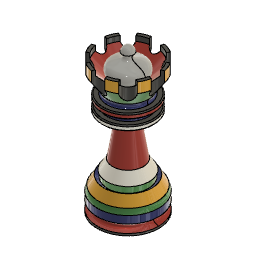
IRFAN NAUFAL CHESSPIECE EA v1 (Autodesk Fusion 360 design; units mm, degrees)
Autodesk Fusion 360 part; units mm, degrees
sketch "Sketch1" plane through (0, 0, 0) normal (0, 1, 0) x (1, 0, 0)
  line L0 (0, 0) -> (0, -140.5)
  line L1 (0, 0) -> (30, 0)
  line L2 (20.255, -85) -> (24.255, -85)
  line L3 (25.255, -86) -> (25.255, -89)
  line L4 (24.255, -90) -> (20.255, -90)
  line L5 (20.255, -90) -> (20.255, -95)
  line L6 (20.255, -95) -> (24.255, -95)
  line L7 (25.255, -96) -> (25.255, -99)
  line L8 (24.255, -100) -> (20.255, -100)
  line L9 (15, -45) -> (10, -75)
  spline S0 degree 5 poles (10, -75) (10.0092, -75.3857) (10.0449, -76.1408) (10.1499, -77.2245) (10.3948, -78.5701) (10.8875, -80.0753) (11.583, -81.3881) (12.4976, -82.4932) (13.6392, -83.3832) (14.9977, -84.0674) (16.5565, -84.5619) (17.9504, -84.8182) (19.0731, -84.9371) (19.8554, -84.9844) (20.255, -85) knots 0 0 0 0 0 0 0.1 0.2 0.3 0.4 0.5 0.6 0.7 0.8 0.9 1 1 1 1 1 1
  line L10 (20.255, -104.758) -> (30, -120)
  line L11 (30, -120) -> (30, -130)
  line L12 (30, -130) -> (27, -130)
  line L13 (27, -130) -> (27, -125)
  line L14 (27, -125) -> (13.4752, -111.6935)
  spline S1 degree 5 poles (20.255, -100) (20.1529, -100.0131) (19.9584, -100.047) (19.6954, -100.1209) (19.4032, -100.2666) (19.1413, -100.5318) (18.9896, -100.8856) (18.9526, -101.3317) (19.0262, -101.8667) (19.2009, -102.4829) (19.4662, -103.172) (19.7438, -103.776) (19.9863, -104.2565) (20.163, -104.5888) (20.255, -104.758) knots 0 0 0 0 0 0 0.1 0.2 0.3 0.4 0.5 0.6 0.7 0.8 0.9 1 1 1 1 1 1
  spline S2 degree 5 poles (13.4752, -111.6935) (13.9081, -112.3459) (14.7093, -113.6174) (15.717, -115.4243) (16.6695, -117.6315) (17.1977, -120.0473) (17.0609, -122.1156) (16.279, -123.8403) (14.9094, -125.2409) (13.0673, -126.3609) (10.941, -127.2753) (8.7579, -128.0759) (6.758, -128.8603) (5.1638, -129.7195) (4.1546, -130.7276) (3.828, -131.9266) (4.1394, -133.0514) (4.6952, -133.9893) (5.208, -134.6562) (5.5, -135) knots 0 0 0 0 0 0 0.066667 0.133333 0.2 0.266667 0.333333 0.4 0.466667 0.533333 0.6 0.666667 0.733333 0.8 0.866667 0.933333 1 1 1 1 1 1
  arc A0 (0, -140.5) -> (5.5, -135) centre (0, -135) ccw
  spline S3 degree 5 poles (30, -1.9966) (29.6151, -2.0924) (28.8795, -2.2899) (27.8789, -2.6032) (26.7537, -3.0558) (25.7187, -3.6835) (25.0859, -4.3783) (24.8847, -5.1451) (25.1244, -5.9854) (25.7808, -6.8952) (26.8192, -7.8688) (27.9291, -8.6942) (28.9084, -9.3377) (29.6254, -9.7775) (30, -10) knots 0 0 0 0 0 0 0.1 0.2 0.3 0.4 0.5 0.6 0.7 0.8 0.9 1 1 1 1 1 1
  line L15 (30, 0) -> (30, -1.9966)
  line L16 (30, -10) -> (30, -17.2302)
  line L17 (20.8586, -35.2357) -> (20, -29)
  line L18 (20, -29) -> (23.3824, -31.0294)
  line L19 (28.5749, -22.3751) -> (23.3824, -31.0294)
  line L20 (20.8586, -35.2357) -> (15, -45)
  arc A1 (28.5749, -22.3751) -> (30, -17.2302) centre (20, -17.2302) ccw
  arc A2 (24.255, -100) -> (25.255, -99) centre (24.255, -99) ccw
  arc A3 (25.255, -96) -> (24.255, -95) centre (24.255, -96) ccw
  arc A4 (24.255, -90) -> (25.255, -89) centre (24.255, -89) ccw
  arc A5 (25.255, -86) -> (24.255, -85) centre (24.255, -86) ccw
  point P0 (12.5, -82.3864)
  point P1 (19, -101)
  point P2 (15, -125)
  point P3 (5, -130)
  point P4 (25, -5)
  dimension "d2" = 11
  dimension "d3" = 10
  dimension "d4" = 1
  constraint coincident L0.start L1.start
  constraint vertical L0
  constraint perpendicular L0 L1
  constraint perpendicular L1 L15
  constraint horizontal L2
  constraint perpendicular L2 L3
  constraint perpendicular L3 L4
  constraint perpendicular L4 L5
  constraint perpendicular L5 L6
  constraint perpendicular L6 L7
  constraint perpendicular L7 L8
  constraint vertical L11
  constraint perpendicular L11 L12
  constraint perpendicular L12 L13
  constraint coincident L0 A0.centre
  constraint collinear L15 L16
  constraint coincident S3.end L15
  constraint coincident L17.start L19
  constraint perpendicular L18 L19
  constraint collinear L19 L20
  constraint tangent L16 A1
  constraint tangent L19 A1
  constraint tangent L7 A2
  constraint tangent L8 A2
  constraint tangent L6 A3
  constraint tangent L7 A3
  constraint equal A2 A3
  constraint tangent L3 A4
  constraint tangent L4 A4
  constraint equal A2 A4
  constraint tangent L2 A5
  constraint tangent L3 A5
  constraint equal A2 A5
  measures "d2" diameter of A0
  measures "d3" radius of A1
  measures "d4" radius of A2
revolve "Revolve1" add sketch "Sketch1" angle 360 about axis through (0, 0, 0) along (0, 0, 1)
sketch "Sketch2" plane through (0, 0, 130) normal (0, 0, 1) x (-1, 0, 0)
  circle A0 centre (0, 0) radius 30
  circle A1 centre (0, 0) radius 27
  circle A2 centre (-30, 0) radius 6.5
  circle A3 centre (0, -30) radius 6.5
  circle A4 centre (30, 0) radius 6.5
  circle A5 centre (0, 30) radius 6.5
  circle A6 centre (21.2132, -21.2132) radius 6.5
  circle A7 centre (30, 0) radius 6.5
  circle A8 centre (21.2132, 21.2132) radius 6.5
  circle A9 centre (0, 30) radius 6.5
  circle A10 centre (-21.2132, 21.2132) radius 6.5
  circle A11 centre (-30, 0) radius 6.5
  circle A12 centre (-21.2132, -21.2132) radius 6.5
  dimension "d6" = 13
  dimension "d7" = 13
  dimension "d8" = 13
  dimension "d9" = 13
  dimension "d15" = 360
  constraint coincident A0 A2.centre
  constraint coincident A0 A3.centre
  constraint coincident A0 A4.centre
  constraint coincident A0 A5.centre
  measures "d6" diameter of A2
  measures "d7" diameter of A3
  measures "d8" diameter of A4
  measures "d9" diameter of A5
extrude "Extrude1" cut sketch "Sketch2" against normal blind 21 contours A0 A1 A2 A11 | A0 A2 A11 | A1 A2 A11
extrude "Extrude2" cut sketch "Sketch2" against normal blind 22 contours A0 A1 A10 | A0 A10 | A1 A10
extrude "Extrude3" cut sketch "Sketch2" against normal blind 25 contours A0 A1 A4 A7 | A0 A4 A7 | A0 A1 A8 | A0 A8 | A1 A4 A7 | A0 A6 | A0 A1 A6 | A1 A8 | A1 A6 | A0 A1 A5 A9 | A0 A5 A9 | A0 A3 | A0 A1 A3 | A1 A5 A9 | A1 A3 | A0 A12 | A0 A1 A12 | A1 A12
